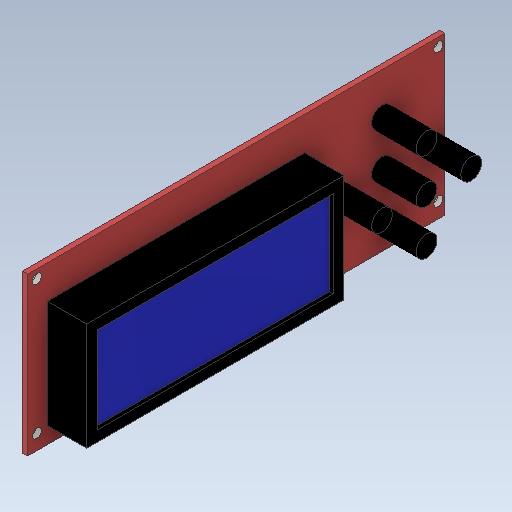
# Autodesk Inventor part: 27_LCD
Saved by Autodesk Inventor 2020.2 (Build 242310000, 310)
## iProperties
Created: 2017-10-29
Part Number: 27_LCD
Material: Ogólny
Document SubType Name: Modeling
Designer: wojte
Density: 1 g/cm^3
Appearance: Domyślna
Author: wojte
Autodesk Inventor part; units mm, degrees
ref_plane "YZ Plane" through (0, 0, 0) normal (1, 0, 0) x (0, 1, 0)
ref_plane "XZ Plane" through (0, 0, 0) normal (0, 1, 0) x (-1, 0, 0)
ref_plane "XY Plane" through (0, 0, 0) normal (0, 0, 1) x (1, 0, 0)
sketch "Szkic1" plane through (0, 0, 0) normal (1, 0, 0) x (0, 1, 0)
  line L0 (0, 0) -> (41, 0)
  line L1 (41, 0) -> (41, -98)
  line L2 (41, -98) -> (0, -98)
  line L3 (0, -98) -> (0, 0)
  dimension "d0" = 98
  dimension "d1" = 41
  constraints: 8 end point, 2 parallel, 1 horizontal, 1 perpendicular
  measures "d0" distance of L2.end L0.start
  measures "d1" distance of L0.start L0.end
extrude "Wyciągnięcie proste1" add sketch "Szkic1" along normal blind 15
sketch "Szkic2" plane through (15, 0, 0) normal (1, 0, 0) x (0, 0, -1)
  line L0 (4, 4) -> (94, 4)
  line L1 (94, 4) -> (94, 37)
  line L2 (94, 37) -> (4, 37)
  line L3 (4, 37) -> (4, 4)
  line L4 (49, 37) -> (49, 41) construction
  line L5 (98, 41) -> (0, 41) projected
  line L6 (94, 20.5) -> (98, 20.5) construction
  line L7 (98, 0) -> (98, 41) projected
  point P0 (0, 0)
  dimension "d4" = 90
  dimension "d5" = 33
  constraints: 12 end point, 4 midpoint, 2 horizontal, 2 parallel, 1 perpendicular, 1 vertical
  measures "d4" distance of L1.end L2.end
  measures "d5" distance of L0.end L1.end
extrude "Wyciągnięcie proste2" cut sketch "Szkic2" against normal blind 1.5
sketch "Szkic3" plane through (0, 0, 0) normal (-1, 0, 0) x (0, 0, 1)
  line L0 (-151.5, 53.7) -> (7.5, 53.7)
  line L1 (7.5, 53.7) -> (7.5, -6.3)
  line L2 (7.5, -6.3) -> (-151.5, -6.3)
  line L3 (-151.5, -6.3) -> (-151.5, 53.7)
  line L4 (-98, 41) -> (0, 41) projected
  line L5 (0, 41) -> (0, 0) projected
  line L6 (-98, 0) -> (0, 0) projected
  dimension "d8" = 159
  dimension "d9" = 60
  dimension "d10" = 7.5
  dimension "d11" = 6.3
  constraints: 8 end point, 2 parallel, 1 horizontal, 1 perpendicular
  measures "d8" distance of L1.end L2.end
  measures "d9" distance of L0.end L1.end
  measures "d10" distance between parallel lines of L1 L5
  measures "d11" distance between parallel lines of L2 L6
extrude "Wyciągnięcie proste3" add sketch "Szkic3" along normal blind 2
sketch "Szkic4" plane through (0, 0, 0) normal (1, 0, 0) x (0, 0, -1)
  line L0 (110.5, 21) -> (144.5, 21) construction
  line L1 (127.5, 4) -> (127.5, 38) construction
  line L2 (98, 40.528) -> (98, -0.472) construction
  line L3 (98, 0) -> (98, 41) projected
  line L4 (0, 0) -> (98, 0) projected
  circle A0 centre (127.5, 38) radius 4
  circle A1 centre (110.5, 21) radius 4
  circle A2 centre (144.5, 21) radius 4
  circle A3 centre (127.5, 4) radius 4
  circle A4 centre (127.5, 21) radius 4
  dimension "d14" = 34
  dimension "d15" = 34
  dimension "d16" = 29.5
  dimension "d17" = 4
  dimension "d18" = 8
  constraints: 9 coincident, 6 end point, 5 centre point, 4 equal radius, 2 symmetric about line, 1 collinear, 1 horizontal, 1 midpoint, 1 vertical
  measures "d14" distance of L0.start L0.end
  measures "d15" distance of L1.start L1.end
  measures "d16" distance between parallel lines of L1 L2
  measures "d17" distance from line of point (127.5, 4) L4
  measures "d18" diameter of A0
sketch "Szkic5" plane through (0, 0, 0) normal (1, 0, 0) x (0, 0, -1)
  line L0 (-4, -0.5) -> (149, -0.5) construction
  line L1 (149, -0.5) -> (149, 50.5) construction
  line L2 (149, 50.5) -> (-4, 50.5) construction
  line L3 (-4, 50.5) -> (-4, -0.5) construction
  line L4 (0, 41) -> (0, 0) projected
  line L5 (0, 0) -> (98, 0) projected
  dimension "d21" = 51
  dimension "d22" = 153
  dimension "d23" = 4
  dimension "d24" = 0.5
  constraints: 8 end point, 4 coincident, 2 parallel, 1 horizontal, 1 perpendicular
  measures "d21" distance of L2.end L0.start
  measures "d22" distance of L0.start L0.end
  measures "d23" distance between parallel lines of L3 L4
  measures "d24" distance between parallel lines of L5 L0
hole "Otwór1" at (0, -0.5, -149) at (0, 50.5, -149) at (0, 50.5, 4) at (0, -0.5, 4) direction (-1, 0, 0) diameter 3.5 end through all
extrude "Wyciągnięcie proste5" add sketch "Szkic4" along normal blind 17
